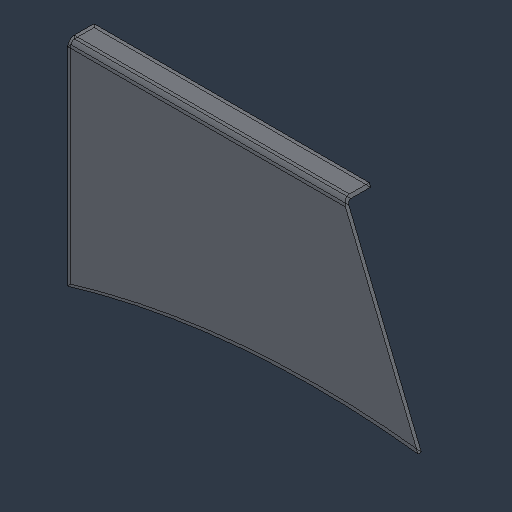
# Autodesk Inventor part: SIDE_INTAKE_LEXAN
Saved by Autodesk Inventor 2026 (Build 300175050, 175E)
## iProperties
Created: 2026-04-02
Part Number: SIDE_INTAKE_LEXAN
Material: Polycarbonate, PC 1000, Clear
Document SubType Name: Sheet Metal
Designer: 4aida
Density: 1.20131 g/cm^3
Sheet Metal Rule: Default_mm
Appearance: Lexan (Clear)
Flat Pattern Width: 22.5986 cm
Flat Pattern Length: 33.7391 cm
Flat Pattern Area: 762.458 cm^2
Sheet Metal Width: 225.986 mm
Sheet Metal Length: 337.391 mm
Sheet Metal Area: 76245.758 mm^2
Mass: 227.73 g
Surface Area: 1227.34 cm^2
Volume: 189.568 cm^3
Author: 4aida
Autodesk Inventor part; units mm, degrees
note: some values were not read from the file. Chosen so that the rebuilt part matches the saved one: flange form of "Plate1".
ref_plane "YZ Plane" through (0, 0, 0) normal (1, 0, 0) x (0, 1, 0)
ref_plane "XZ Plane" through (0, 0, 0) normal (0, 1, 0) x (-1, 0, 0)
ref_plane "XY Plane" through (0, 0, 0) normal (0, 0, 1) x (1, 0, 0)
sketch "Sketch1" plane through (0, 0, 0) normal (1, 0, 0) x (0, 1, 0)
  line L0 (0, 0) -> (250, 0)
  line L1 (250, 0) -> (250, -25.4)
  dimension "d0" = 25.4
  dimension "d1" = 250
  measures "d0" distance of L0.end L1.end
  measures "d1" distance of L0.start L0.end
contour flange "Contour Flange1" sketch "Sketch1" thickness 3.175 bend radius 3.175 width 350 along (1, 0, 0) mid plane no both sides no wall seen from (0, 125, 0) lies toward (0, 0, -1) curves L0 L1
bend "Bend1"
corner "Corner1"
sketch "Sketch2" plane through (0, 0, 0) normal (0, 0, 1) x (1, 0, 0)
  line L0 (350, 0) -> (350, 243.65) projected
  line L1 (0, 0) -> (0, 243.65) projected
  line L2 (0, 243.65) -> (350, 243.65) projected
  line L3 (0, 0) -> (0, 243.65) projected
  line L4 (350, 0) -> (0, 0) projected
  line L5 (350, 243.65) -> (350, 0) projected
  arc A0 (269.2821, 77.9424) -> (167.772, 75.6113) centre (237.5885, -753.3037) ccw
  arc A1 (167.772, 75.6113) -> (0, 43.8953) centre (237.5885, -753.3037) ccw
  arc A2 (350, 70.916) -> (269.2821, 77.9424) centre (237.5885, -753.3037) ccw
  point P0 (0, 61.7144)
  point P1 (350, 0)
  point P2 (350, 70.916)
  point P3 (0, 43.8953)
  constraints: 6 point on circle, 4 concentric, 3 centre point, 3 point on line, 4 other
extrude "Cut1" cut sketch "Sketch2" against normal blind 3.175 contours L4 L1 A1 A0 A2 L0
sketch "Sketch7" plane through (0, 243.65, 0) normal (0, 0, 1) x (1, 0, 0)
  line L0 (350, 0) -> (350, -172.734) construction
  line L1 (0, 0) -> (350, 0) construction
  line L2 (0, -199.7547) -> (0, 0) construction
  line L3 (350, -202.0252) -> (265.0055, 6.35)
  line L4 (0, 6.35) -> (350, 6.35) construction
  line L5 (350, -202.0252) -> (350, 6.35)
  line L6 (350, 6.35) -> (265.0055, 6.35)
  arc A0 (350, -172.734) -> (0, -199.7547) centre (237.5885, -996.9537) ccw projected
  point P0 (0, -243.65)
  point P1 (346.825, 6.35)
  dimension "d56" = 22.19
  constraints: 6 end point, 2 point on line, 1 perpendicular, 1 vertical
  measures "d56" angle of L0 L3
extrude "Cut4" cut sketch "Sketch7" along normal through all both and the other way through all
equation "\"d14\" = Thickness"
equation "\"d57\" = Thickness"
equation "\"d2\" = Thickness"
equation "\"d3\" = BendReliefWidth"
equation "\"d4\" = BendReliefDepth"
equation "\"d5\" = MinimumRemnant"
equation "\"d6\" = TransitionRadius"
equation "\"d8\" = BendRadius"
equation "\"d10\" = CornerReliefSize"
equation "\"d11\" = GapSize"
equation "\"d12\" = JacobiRadiusSize"
equation "\"BendRadius\" = Thickness"
equation "\"BendReliefWidth\" = Thickness"
equation "\"BendReliefDepth\" = 0.5 * Thickness"
equation "\"CornerReliefSize\" = 4 * Thickness"
equation "\"MinimumRemnant\" = 2 * Thickness"
equation "\"TransitionRadius\" = BendRadius"
equation "\"JacobiRadiusSize\" = BendRadius"
equation "\"GapSize\" = Thickness"
equation "\"Thickness\" = 3.175"
body "Solid1"
